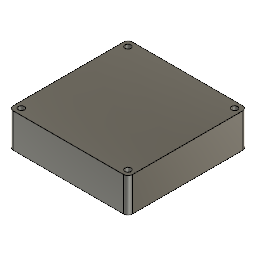
2024-12-28.2_development_hexapod_mounts (Autodesk Fusion 360 archive; units mm, degrees)
design "noctua_fan_80mm"
Autodesk Fusion 360 part; units mm, degrees
(part 1 of 2)
box "BoxPrimitive1" add length 80 width 80 height 23 placed x (0, -1, 0) y (1, 0, 0) z (0, 0, 1) at (0, 0, 0)
fillet "Fillet1" radius 3 4 edges at (0, -80, 11.5) (80, -80, 11.5) (80, 0, 11.5) (0, 0, 11.5)
sketch "Sketch2" plane through (0, 0, 23) normal (0, 0, 1) x (-1, 0, 0)
  arc A0 (-3, 0) -> (0, 3) centre (-3, 3) ccw
  line L0 (0, 3) -> (0, 77)
  arc A1 (0, 77) -> (-3, 80) centre (-3, 77) ccw
  line L1 (-3, 80) -> (-77, 80)
  arc A2 (-77, 80) -> (-80, 77) centre (-77, 77) ccw
  line L2 (-80, 77) -> (-80, 3)
  arc A3 (-80, 3) -> (-77, 0) centre (-77, 3) ccw
  line L3 (-77, 0) -> (-3, 0)
  circle A4 centre (-75.75, 75.75) radius 2
  circle A5 centre (-75.75, 4.25) radius 2
  circle A6 centre (-4.25, 75.75) radius 2
  circle A7 centre (-4.25, 4.25) radius 2
  dimension "d8" = 4
  dimension "d9" = 4
  dimension "d10" = 4
  dimension "d11" = 4
  dimension "d12" = 4.25
  dimension "d13" = 4.25
  dimension "d14" = 4.25
  dimension "d15" = 4.25
  dimension "d16" = 4.25
  dimension "d17" = 4.25
  dimension "d18" = 4.25
  dimension "d19" = 4.25
  measures "d8" diameter of A4
  measures "d9" diameter of A5
  measures "d10" diameter of A6
  measures "d11" diameter of A7
  measures "d12" distance of L1 A4.centre
  measures "d13" distance of L2 A4.centre
  measures "d14" distance of L3 A5.centre
  measures "d15" distance of L2 A5.centre
  measures "d16" distance of L3 A7.centre
  measures "d17" distance of L0 A7.centre
  measures "d18" distance of L1 A6.centre
  measures "d19" distance of L0 A6.centre
extrude "Extrude1" cut sketch "Sketch2" against normal blind 35 contours A4 | A5 | A6 | A7

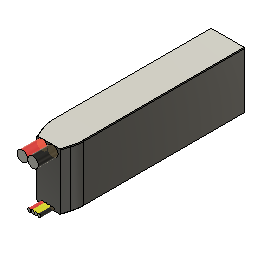
design "battery"
Autodesk Fusion 360 part; units mm, degrees
sketch "Sketch1" plane through (0, 0, 0) normal (0, 0, 1) x (1, 0, 0)
  line L0 (0, 0) -> (26, 0)
  line L1 (26, 0) -> (26, 137)
  line L2 (26, 137) -> (0, 137)
  line L3 (0, 137) -> (0, 0)
  dimension "d1" = 26
  dimension "d2" = 137
  constraint horizontal L0
  constraint vertical L1
  constraint horizontal L2
  constraint vertical L3
  constraint coincident L0.start L3.end
  measures "d1" distance of L0.start L0.end
  measures "d2" distance of L0.start L2.end
extrude "Extrude1" add sketch "Sketch1" along normal blind 43 makes body 1
sketch "Sketch2" plane through (0, 0, 0) normal (0, -1, 0) x (1, 0, 0)
  line L0 (0, 0) -> (26, 0)
  line L1 (26, 0) -> (26, 43)
  line L2 (26, 43) -> (0, 43)
  line L3 (0, 43) -> (0, 0)
  line L4 (21, 35) -> (5, 35) construction
  line L5 (5, 35) -> (5, 51) construction
  line L6 (5, 51) -> (21, 51) construction
  line L7 (21, 51) -> (21, 35) construction
  line L8 (21, 35) -> (5, 51) construction
  line L9 (5, 35) -> (21, 51) construction
  line L10 (13, 43) -> (5, 35) construction
  line L11 (13, 43) -> (21, 35) construction
  circle A0 centre (9, 39) radius 4
  circle A1 centre (17, 39) radius 4
  point P0 (13, 43)
  dimension "d5" = 16
  dimension "d6" = 16
  constraint horizontal L4
  constraint perpendicular L4 L5
  constraint parallel L4 L6
  constraint parallel L5 L7
  constraint coincident L8 P0
  constraint coincident L9 P0
  constraint midpoint L2 P0
  constraint coincident P0 L10.start
  constraint midpoint L10 A0.centre
  constraint tangent L2 A0
  constraint midpoint L11 A1.centre
  constraint tangent L2 A1
  measures "d5" distance of L5.end L6.end
  measures "d6" distance of L4.end L5.end
extrude "Extrude2" add sketch "Sketch2" along normal blind 15 separate body contours A0 | A1 makes body 2
sketch "Sketch3" plane through (0, 0, 0) normal (0, -1, 0) x (1, 0, 0)
  line L0 (0, 0) -> (26, 0)
  line L1 (26, 0) -> (26, 43)
  line L2 (26, 43) -> (0, 43)
  line L3 (0, 43) -> (0, 0)
  line L4 (18, 2.5) -> (8, 2.5) construction
  line L5 (8, 2.5) -> (8, -2.5) construction
  line L6 (8, -2.5) -> (18, -2.5) construction
  line L7 (18, -2.5) -> (18, 2.5) construction
  line L8 (18, 2.5) -> (8, -2.5) construction
  line L9 (8, 2.5) -> (18, -2.5) construction
  line L10 (8, 2.5) -> (8, 0)
  line L11 (8, 1.25) -> (9.25, 1.25) construction
  circle A0 centre (9.25, 1.25) radius 1.25
  circle A1 centre (11.75, 1.25) radius 1.25
  circle A2 centre (14.25, 1.25) radius 1.25
  circle A3 centre (16.75, 1.25) radius 1.25
  point P0 (13, 0)
  dimension "d9" = 10
  dimension "d10" = 5
  dimension "d11" = 1.25
  constraint horizontal L4
  constraint perpendicular L4 L5
  constraint parallel L4 L6
  constraint parallel L5 L7
  constraint coincident L8 P0
  constraint coincident L9 P0
  constraint midpoint L0 P0
  constraint midpoint L5 L10.end
  constraint midpoint L10 L11.start
  constraint perpendicular L5 L11
  constraint coincident L11.end A0.centre
  constraint tangent L4 A0
  measures "d9" distance of L5.end L6.end
  measures "d10" distance of L4.end L5.end
  measures "d11" distance of L11.start L11.end
extrude "Extrude3" add sketch "Sketch3" along normal blind 10 separate body contours A0 | A1 | A2 | A3 makes body 3
chamfer "Chamfer1" distance 3 distance2 10 1 edges at (26, 0, 21.5) measured on face at (8.6667, 0, 14.3333) on bodies 1
chamfer "Chamfer2" distance 12 distance2 5 1 edges at (0, 0, 21.5) measured on face at (0, 91.3333, 14.3333) on bodies 1
fillet "Fillet1" radius 30 2 edges at (0, 12, 21.5) (26, 10, 21.5) on bodies 1
chamfer "Chamfer3" distance 0.5 distance2 0.5 12 edges at (25.682, 10.0467, 0) (26, 75.7015, 0) (23.8674, 2.8913, 0) (0, 77.5, 0) (0.5826, 12.1165, 0) (3.6538, 3.2308, 0) (0.5826, 12.1165, 43) (0, 77.5, 43) (3.6538, 3.2308, 43) (26, 75.7015, 43) (23.8674, 2.8913, 43) (25.682, 10.0467, 43) 1 faces at (17.3333, 137, 14.3333) measured on face at (25.9843, 13.4317, 14.3333) measured on face at (26, 55.2687, 14.3333) measured on face at (23.5783, 1.9275, 14.3333) measured on face at (0, 97.3333, 14.3333) measured on face at (1.8284, 7.687, 28.6667) measured on face at (3.2051, 4.3077, 28.6667) measured on face at (1.8284, 7.687, 28.6667) measured on face at (17.3333, 56.4677, 43) measured on face at (3.2051, 4.3077, 28.6667) measured on face at (17.3333, 56.4677, 43) measured on face at (23.5783, 1.9275, 14.3333) measured on face at (25.9843, 13.4317, 14.3333) on bodies 1

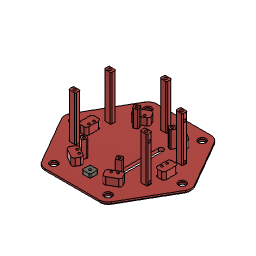
design "base"
Autodesk Fusion 360 part; units mm, degrees
sketch "Sketch1" plane through (0, 0, 0) normal (0, 0, 1) x (1, 0, 0)
  line L0 (130, 0) -> (65, 112.5833)
  line L1 (65, 112.5833) -> (-65, 112.5833)
  line L2 (-65, 112.5833) -> (-130, 0)
  line L3 (-130, 0) -> (-65, -112.5833)
  line L4 (-65, -112.5833) -> (65, -112.5833)
  line L5 (65, -112.5833) -> (130, 0)
  dimension "d1" = 130
  measures "d1" distance of L0.start origin
extrude "Extrude1" add sketch "Sketch1" along normal blind 6.5 makes body 1
fillet "Fillet1" radius 18 6 edges at (-130, 0, 3.25) (-65, -112.5833, 3.25) (65, -112.5833, 3.25) (130, 0, 3.25) (65, 112.5833, 3.25) (-65, 112.5833, 3.25) on bodies 1
chamfer "Chamfer2" distance 3.25 angle 45 12 edges at (0, -112.5833, 0) (63.6077, -110.1718, 0) (97.5, -56.2917, 0) (127.2154, 0, 0) (97.5, 56.2917, 0) (63.6077, 110.1718, 0) (0, 112.5833, 0) (-63.6077, 110.1718, 0) (-97.5, 56.2917, 0) (-127.2154, 0, 0) (-97.5, -56.2917, 0) (-63.6077, -110.1718, 0) on bodies 1
sketch "Sketch2" plane through (0, 0, 6.5) normal (0, 0, 1) x (-1, 0, 0)
  arc A0 (54.6077, -112.5833) -> (70.1962, -103.5833) centre (54.6077, -94.5833) ccw
  line L0 (70.1962, -103.5833) -> (124.8038, -9)
  arc A1 (124.8038, -9) -> (124.8038, 9) centre (109.2154, 0) ccw
  line L1 (124.8038, 9) -> (70.1962, 103.5833)
  line L2 (54.6077, 112.5833) -> (-54.6077, 112.5833)
  line L3 (-70.1962, 103.5833) -> (-124.8038, 9)
  arc A2 (-124.8038, 9) -> (-124.8038, -9) centre (-109.2154, 0) ccw
  line L4 (-124.8038, -9) -> (-70.1962, -103.5833)
  arc A3 (-70.1962, -103.5833) -> (-54.6077, -112.5833) centre (-54.6077, -94.5833) ccw
  line L5 (-54.6077, -112.5833) -> (54.6077, -112.5833)
  circle A4 centre (109.2154, 0) radius 7
  circle A5 centre (109.2154, 0) radius 6
  circle A6 centre (73.4654, -5) radius 2.25
  arc A7 (73.7154, 14.55) -> (68.7154, 9.55) centre (73.7154, 9.55) ccw
  line L6 (68.7154, 9.55) -> (68.7154, -9.55)
  circle A8 centre (73.4654, 5) radius 2.25
  line L7 (86.7154, 9.55) -> (86.7154, -9.55)
  line L8 (68.7154, 0) -> (86.7154, 0) construction
  arc A9 (68.7154, -9.55) -> (73.7154, -14.55) centre (73.7154, -9.55) ccw
  arc A10 (73.7154, 14.55) -> (68.7154, 9.55) centre (73.7154, 9.55) ccw
  line L9 (81.7154, 14.55) -> (73.7154, 14.55)
  line L10 (73.7154, -14.55) -> (81.7154, -14.55)
  line L11 (73.4654, 5) -> (68.7154, 5) construction
  line L12 (73.4654, -5) -> (68.7154, -5) construction
  line L13 (127.2154, 0) -> (-127.2154, 0) construction
  line L14 (0, -112.5833) -> (0, 112.5833) construction
  arc A11 (-124.8038, 9) -> (-124.8038, -9) centre (-109.2154, 0) ccw
  arc A12 (-70.1962, -103.5833) -> (-54.6077, -112.5833) centre (-54.6077, -94.5833) ccw
  arc A13 (54.6077, -112.5833) -> (70.1962, -103.5833) centre (54.6077, -94.5833) ccw
  arc A14 (81.7154, -14.55) -> (86.7154, -9.55) centre (81.7154, -9.55) ccw
  arc A15 (86.7154, 9.55) -> (81.7154, 14.55) centre (81.7154, 9.55) ccw
  circle A16 centre (32.4026, 66.1229) radius 2.25
  line L15 (34.3577, 59.5093) -> (43.3577, 75.0977) construction
  arc A17 (70.1962, 103.5833) -> (54.6077, 112.5833) centre (54.6077, 94.5833) ccw
  arc A18 (42.6282, 54.7343) -> (49.4584, 56.5644) centre (45.1282, 59.0644) ccw
  line L16 (41.0628, 61.1229) -> (38.6878, 57.0093) construction
  arc A19 (24.257, 71.1144) -> (26.0872, 64.2843) centre (28.5872, 68.6144) ccw
  line L17 (28.257, 78.0426) -> (24.257, 71.1144)
  circle A20 centre (41.0628, 61.1229) radius 2.25
  arc A21 (53.4584, 63.4926) -> (51.6282, 70.3227) centre (49.1282, 65.9926) ccw
  circle A22 centre (54.6077, 94.5833) radius 6
  circle A23 centre (54.6077, 94.5833) radius 7
  line L18 (32.4026, 66.1229) -> (30.0276, 62.0093) construction
  arc A24 (24.257, 71.1144) -> (26.0872, 64.2843) centre (28.5872, 68.6144) ccw
  line L19 (26.0872, 64.2843) -> (42.6282, 54.7343)
  line L20 (49.4584, 56.5644) -> (53.4584, 63.4926)
  line L21 (35.0872, 79.8727) -> (51.6282, 70.3227)
  arc A25 (35.0872, 79.8727) -> (28.257, 78.0426) centre (32.5872, 75.5426) ccw
  circle A26 centre (-41.0628, 61.1229) radius 2.25
  line L22 (-42.6282, 54.7343) -> (-26.0872, 64.2843)
  line L23 (-34.3577, 59.5093) -> (-43.3577, 75.0977) construction
  arc A27 (-54.6077, 112.5833) -> (-70.1962, 103.5833) centre (-54.6077, 94.5833) ccw
  arc A28 (-26.0872, 64.2843) -> (-24.257, 71.1144) centre (-28.5872, 68.6144) ccw
  line L24 (-32.4026, 66.1229) -> (-30.0276, 62.0093) construction
  arc A29 (-49.4584, 56.5644) -> (-42.6282, 54.7343) centre (-45.1282, 59.0644) ccw
  line L25 (-53.4584, 63.4926) -> (-49.4584, 56.5644)
  circle A30 centre (-32.4026, 66.1229) radius 2.25
  arc A31 (-28.257, 78.0426) -> (-35.0872, 79.8727) centre (-32.5872, 75.5426) ccw
  circle A32 centre (-54.6077, 94.5833) radius 6
  circle A33 centre (-54.6077, 94.5833) radius 7
  line L26 (-41.0628, 61.1229) -> (-38.6878, 57.0093) construction
  arc A34 (-49.4584, 56.5644) -> (-42.6282, 54.7343) centre (-45.1282, 59.0644) ccw
  line L27 (-42.6282, 54.7343) -> (-26.0872, 64.2843)
  line L28 (-24.257, 71.1144) -> (-28.257, 78.0426)
  line L29 (-51.6282, 70.3227) -> (-35.0872, 79.8727)
  arc A35 (-51.6282, 70.3227) -> (-53.4584, 63.4926) centre (-49.1282, 65.9926) ccw
  circle A36 centre (-73.4654, -5) radius 2.25
  line L30 (-68.7154, -9.55) -> (-68.7154, 9.55)
  line L31 (-68.7154, 0) -> (-86.7154, 0) construction
  arc A37 (-124.8038, 9) -> (-124.8038, -9) centre (-109.2154, 0) ccw
  arc A38 (-68.7154, 9.55) -> (-73.7154, 14.55) centre (-73.7154, 9.55) ccw
  line L32 (-73.4654, 5) -> (-68.7154, 5) construction
  arc A39 (-73.7154, -14.55) -> (-68.7154, -9.55) centre (-73.7154, -9.55) ccw
  line L33 (-81.7154, -14.55) -> (-73.7154, -14.55)
  circle A40 centre (-73.4654, 5) radius 2.25
  arc A41 (-81.7154, 14.55) -> (-86.7154, 9.55) centre (-81.7154, 9.55) ccw
  circle A42 centre (-109.2154, 0) radius 6
  circle A43 centre (-109.2154, 0) radius 7
  line L34 (-73.4654, -5) -> (-68.7154, -5) construction
  arc A44 (-73.7154, -14.55) -> (-68.7154, -9.55) centre (-73.7154, -9.55) ccw
  line L35 (-68.7154, -9.55) -> (-68.7154, 9.55)
  line L36 (-73.7154, 14.55) -> (-81.7154, 14.55)
  line L37 (-86.7154, -9.55) -> (-86.7154, 9.55)
  arc A45 (-86.7154, -9.55) -> (-81.7154, -14.55) centre (-81.7154, -9.55) ccw
  circle A46 centre (-32.4026, -66.1229) radius 2.25
  line L38 (-26.0872, -64.2843) -> (-42.6282, -54.7343)
  line L39 (-34.3577, -59.5093) -> (-43.3577, -75.0977) construction
  arc A47 (-70.1962, -103.5833) -> (-54.6077, -112.5833) centre (-54.6077, -94.5833) ccw
  arc A48 (-42.6282, -54.7343) -> (-49.4584, -56.5644) centre (-45.1282, -59.0644) ccw
  line L40 (-41.0628, -61.1229) -> (-38.6878, -57.0093) construction
  arc A49 (-24.257, -71.1144) -> (-26.0872, -64.2843) centre (-28.5872, -68.6144) ccw
  line L41 (-28.257, -78.0426) -> (-24.257, -71.1144)
  circle A50 centre (-41.0628, -61.1229) radius 2.25
  arc A51 (-53.4584, -63.4926) -> (-51.6282, -70.3227) centre (-49.1282, -65.9926) ccw
  circle A52 centre (-54.6077, -94.5833) radius 6
  circle A53 centre (-54.6077, -94.5833) radius 7
  line L42 (-32.4026, -66.1229) -> (-30.0276, -62.0093) construction
  arc A54 (-24.257, -71.1144) -> (-26.0872, -64.2843) centre (-28.5872, -68.6144) ccw
  line L43 (-26.0872, -64.2843) -> (-42.6282, -54.7343)
  line L44 (-49.4584, -56.5644) -> (-53.4584, -63.4926)
  line L45 (-35.0872, -79.8727) -> (-51.6282, -70.3227)
  arc A55 (-35.0872, -79.8727) -> (-28.257, -78.0426) centre (-32.5872, -75.5426) ccw
  circle A56 centre (41.0628, -61.1229) radius 2.25
  line L46 (34.3577, -59.5093) -> (43.3577, -75.0977) construction
  arc A57 (54.6077, -112.5833) -> (70.1962, -103.5833) centre (54.6077, -94.5833) ccw
  arc A58 (26.0872, -64.2843) -> (24.257, -71.1144) centre (28.5872, -68.6144) ccw
  line L47 (32.4026, -66.1229) -> (30.0276, -62.0093) construction
  arc A59 (49.4584, -56.5644) -> (42.6282, -54.7343) centre (45.1282, -59.0644) ccw
  line L48 (53.4584, -63.4926) -> (49.4584, -56.5644)
  circle A60 centre (32.4026, -66.1229) radius 2.25
  arc A61 (28.257, -78.0426) -> (35.0872, -79.8727) centre (32.5872, -75.5426) ccw
  circle A62 centre (54.6077, -94.5833) radius 6
  circle A63 centre (54.6077, -94.5833) radius 7
  line L49 (41.0628, -61.1229) -> (38.6878, -57.0093) construction
  arc A64 (49.4584, -56.5644) -> (42.6282, -54.7343) centre (45.1282, -59.0644) ccw
  line L50 (42.6282, -54.7343) -> (26.0872, -64.2843)
  line L51 (24.257, -71.1144) -> (28.257, -78.0426)
  line L52 (51.6282, -70.3227) -> (35.0872, -79.8727)
  arc A65 (51.6282, -70.3227) -> (53.4584, -63.4926) centre (49.1282, -65.9926) ccw
  circle A66 centre (73.4654, -5) radius 2.85
  circle A67 centre (73.4654, 5) radius 2.85
  circle A68 centre (41.0628, 61.1229) radius 2.85
  circle A69 centre (32.4026, 66.1229) radius 2.85
  circle A70 centre (-32.4026, 66.1229) radius 2.85
  circle A71 centre (-41.0628, 61.1229) radius 2.85
  circle A72 centre (-73.4654, 5) radius 2.85
  circle A73 centre (-73.4654, -5) radius 2.85
  circle A74 centre (-41.0628, -61.1229) radius 2.85
  circle A75 centre (-32.4026, -66.1229) radius 2.85
  circle A76 centre (32.4026, -66.1229) radius 2.85
  circle A77 centre (41.0628, -61.1229) radius 2.85
  line L53 (-77, -30.6738) -> (-67, -30.6738)
  line L54 (-65, -32.6738) -> (-65, -38.6134)
  line L55 (-67, -40.6134) -> (-77, -40.6134)
  line L56 (-79, -38.6134) -> (-79, -32.6738)
  line L57 (-77, 40.6096) -> (-67, 40.6096)
  line L58 (-65, 38.6096) -> (-65, 32.6738)
  line L59 (-67, 30.6738) -> (-77, 30.6738)
  line L60 (-79, 32.6738) -> (-79, 38.6096)
  line L61 (-72, -35.5) -> (-72, 13.37) construction
  line L62 (-72, 35.5) -> (-72, 30.8281) construction
  circle A78 centre (-72, 35.5) radius 2.85
  circle A79 centre (-72, -35.5) radius 2.85
  arc A80 (-65, -32.6738) -> (-67, -30.6738) centre (-67, -32.6738) ccw
  arc A81 (-67, -40.6134) -> (-65, -38.6134) centre (-67, -38.6134) ccw
  arc A82 (-77, -30.6738) -> (-79, -32.6738) centre (-77, -32.6738) ccw
  arc A83 (-79, -38.6134) -> (-77, -40.6134) centre (-77, -38.6134) ccw
  arc A84 (-67, 30.6738) -> (-65, 32.6738) centre (-67, 32.6738) ccw
  arc A85 (-65, 38.6096) -> (-67, 40.6096) centre (-67, 38.6096) ccw
  arc A86 (-77, 40.6096) -> (-79, 38.6096) centre (-77, 38.6096) ccw
  arc A87 (-79, 32.6738) -> (-77, 30.6738) centre (-77, 32.6738) ccw
  arc A88 (66.7634, -30.6879) -> (65, -32.6738) centre (67, -32.6738) ccw
  arc A89 (77, -40.6134) -> (79, -38.6134) centre (77, -38.6134) ccw
  line L63 (67, -40.6134) -> (77, -40.6134)
  arc A90 (79, -32.6738) -> (77, -30.6738) centre (77, -32.6738) ccw
  line L64 (79, -38.6134) -> (79, -32.6738)
  line L65 (65, -32.6738) -> (65, -38.6134)
  circle A91 centre (72, -35.5) radius 2.85
  arc A92 (65, -38.6134) -> (67, -40.6134) centre (67, -38.6134) ccw
  arc A93 (79, 38.6096) -> (77, 40.6096) centre (77, 38.6096) ccw
  line L66 (77, 40.6096) -> (67, 40.6096)
  arc A94 (77, 30.6738) -> (79, 32.6738) centre (77, 32.6738) ccw
  arc A95 (67, 40.6096) -> (65, 38.6096) centre (67, 38.6096) ccw
  circle A96 centre (72, 35.5) radius 2.85
  arc A97 (65, 32.6738) -> (66.7634, 30.6879) centre (67, 32.6738) ccw
  line L67 (-24, 37.5) -> (-24, -37.5)
  line L68 (-34, -37.5) -> (-34, 37.5)
  line L69 (-34, 40.2042) -> (-24, -40) construction
  line L70 (-24, 40) -> (-34, -40.2042) construction
  line L71 (68.7154, 0) -> (68.7154, 5) construction
  line L72 (63.7154, -5) -> (68.7154, 5) construction
  line L73 (68.7154, -5) -> (63.7154, 5) construction
  line L74 (-42.6282, -54.7343) -> (-26.0872, -64.2843)
  line L75 (42.6282, 54.7343) -> (26.0872, 64.2843)
  line L76 (-42.6282, 54.7343) -> (-26.0872, 64.2843)
  arc A98 (-34, -37.5) -> (-24, -37.5) centre (-29, -37.5) ccw
  arc A99 (-24, 37.5) -> (-34, 37.5) centre (-29, 37.5) ccw
  line L77 (-6, 84.2496) -> (6.5, 84.2496)
  line L78 (8.5, 82.2496) -> (8.5, 69.7496)
  line L79 (6.5, 67.7496) -> (-6, 67.7496)
  line L80 (-8, 69.7496) -> (-8, 82.2496)
  line L81 (-8, 84.2496) -> (8.5, 67.7496) construction
  line L82 (8.5, 84.2496) -> (-8, 67.7496) construction
  arc A100 (6.5, 67.7496) -> (8.5, 69.7496) centre (6.5, 69.7496) ccw
  arc A101 (8.5, 82.2496) -> (6.5, 84.2496) centre (6.5, 82.2496) ccw
  arc A102 (-6, 84.2496) -> (-8, 82.2496) centre (-6, 82.2496) ccw
  arc A103 (-8, 69.7496) -> (-6, 67.7496) centre (-6, 69.7496) ccw
  circle A104 centre (0.25, 75.9996) radius 2.25
  circle A105 centre (0.25, 75.9996) radius 2.85
  circle A106 centre (0, -76) radius 2.85
  line L83 (-5, -71) -> (5, -71)
  line L84 (7, -73) -> (7, -79)
  line L85 (5, -81) -> (-5, -81)
  line L86 (-7, -79) -> (-7, -73)
  line L87 (-7, -71) -> (7, -81) construction
  line L88 (7, -71) -> (-7, -81) construction
  arc A107 (5, -81) -> (7, -79) centre (5, -79) ccw
  arc A108 (7, -73) -> (5, -71) centre (5, -73) ccw
  arc A109 (-5, -71) -> (-7, -73) centre (-5, -73) ccw
  arc A110 (-7, -79) -> (-5, -81) centre (-5, -79) ccw
  line L89 (77, 30.6738) -> (66.7634, 30.6879)
  line L90 (77, -30.6738) -> (66.7634, -30.6879)
  line L91 (65, 32.6738) -> (65, 38.6096)
  line L92 (79, 32.6738) -> (79, 38.6096)
  line L93 (-35.8962, -47.074) -> (-30.7, -50.074)
  line L94 (-29.968, -52.8061) -> (-33.968, -59.7343)
  line L95 (-33.968, -59.7343) -> (-42.6282, -54.7343)
  line L96 (-42.6282, -54.7343) -> (-38.6282, -47.8061)
  line L97 (-37.6282, -46.074) -> (-33.968, -59.7343) construction
  line L98 (-28.968, -51.074) -> (-42.6282, -54.7343) construction
  line L99 (-24.257, -71.1144) -> (-16.5609, -57.7844) construction
  line L100 (-42.6282, -54.7343) -> (-38.8577, -48.2035) construction
  circle A111 centre (-35.7981, -52.9041) radius 2.25
  arc A112 (-29.968, -52.8061) -> (-30.7, -50.074) centre (-31.7, -51.8061) ccw
  arc A113 (-35.8962, -47.074) -> (-38.6282, -47.8061) centre (-36.8962, -48.8061) ccw
  line L101 (-29.968, 52.8061) -> (-33.968, 59.7343)
  line L102 (-35.8962, 47.074) -> (-30.7, 50.074)
  arc A114 (-30.7, 50.074) -> (-29.968, 52.8061) centre (-31.7, 51.8061) ccw
  arc A115 (-38.6282, 47.8061) -> (-35.8962, 47.074) centre (-36.8962, 48.8061) ccw
  line L103 (-42.6282, 54.7343) -> (-38.6282, 47.8061)
  circle A116 centre (-35.7981, 52.9041) radius 2.25
  line L104 (29.968, 52.8061) -> (33.968, 59.7343)
  arc A117 (29.968, 52.8061) -> (30.7, 50.074) centre (31.7, 51.8061) ccw
  line L105 (35.8962, 47.074) -> (30.7, 50.074)
  arc A118 (35.8962, 47.074) -> (38.6282, 47.8061) centre (36.8962, 48.8061) ccw
  line L106 (42.6282, 54.7343) -> (38.6282, 47.8061)
  circle A119 centre (35.7981, 52.9041) radius 2.25
  line L107 (29.968, -52.8061) -> (33.968, -59.7343)
  arc A120 (30.7, -50.074) -> (29.968, -52.8061) centre (31.7, -51.8061) ccw
  line L108 (35.8962, -47.074) -> (30.7, -50.074)
  arc A121 (38.6282, -47.8061) -> (35.8962, -47.074) centre (36.8962, -48.8061) ccw
  line L109 (42.6282, -54.7343) -> (38.6282, -47.8061)
  circle A122 centre (35.7981, -52.9041) radius 2.25
  point P0 (63.6077, 110.1718)
  point P1 (-63.6077, 110.1718)
  point P2 (-127.2154, 0)
  point P3 (-63.6077, -110.1718)
  point P4 (63.6077, -110.1718)
  point P5 (-72, -35.5)
  point P6 (-72, 35.5)
  point P7 (72, -35.5)
  point P8 (72, -35.5)
  point P9 (72, 35.5)
  point P10 (72, 35.5)
  point P11 (-28.9873, 0)
  point P12 (0, 76)
  point P13 (0, 72)
  point P14 (0.25, 75.9996)
  point P15 (0, -76)
  point P16 (-35.7981, -52.9041)
  point P17 (-35.7981, 52.9041)
  dimension "d8" = 14
  dimension "d9" = 12
  dimension "d10" = 18
  dimension "d11" = 9.55
  dimension "d12" = 9.55
  dimension "d15" = 29.1
  dimension "d30" = 5
  dimension "d33" = 4.5
  dimension "d34" = 4.5
  dimension "d35" = 5.7
  dimension "d36" = 5.7
  dimension "d49" = 72
  dimension "d50" = 5.7
  dimension "d51" = 5.7
  dimension "d53" = 2
  dimension "d75" = 35.5
  dimension "d76" = 35.5
  dimension "d78" = 80
  dimension "d79" = 24
  dimension "d84" = 5
  dimension "d85" = 5
  dimension "d86" = 10
  dimension "d135" = 10
  dimension "d164" = 16.5
  dimension "d165" = 16.5
  dimension "d166" = 2
  dimension "d170" = 76
  dimension "d171" = 4.5
  dimension "d172" = 5.7
  dimension "d173" = 5.7
  dimension "d174" = 76
  dimension "d175" = 14
  dimension "d176" = 10
  dimension "d177" = 2
  dimension "d188" = 7
  dimension "d189" = 7
  dimension "d190" = 10
  dimension "d191" = 10
  dimension "d192" = 4.5
  dimension "d193" = 2
  constraint concentric A1 A4
  constraint concentric A4 A5
  constraint coincident A7.end L6.start
  constraint coincident L6.end A9.start
  constraint coincident A9.end L10.start
  constraint coincident A7.start A10.start
  constraint coincident L8.end L7
  constraint parallel L9 L10
  constraint parallel L6 L7
  constraint coincident A8.centre L11.start
  constraint coincident A6.centre L12.start
  constraint midpoint A1 L13.start
  constraint midpoint A2 P2
  constraint midpoint L5 L14.start
  constraint midpoint L2 L14.end
  constraint collinear L8 L13
  constraint tangent L10 A14
  constraint tangent L7 A14
  constraint tangent L7 A15
  constraint tangent L9 A15
  constraint equal A14 A15
  constraint concentric A6 A66
  constraint horizontal L53
  constraint perpendicular L53 L54
  constraint parallel L53 L55
  constraint parallel L54 L56
  constraint horizontal L57
  constraint perpendicular L57 L58
  constraint parallel L57 L59
  constraint parallel L58 L60
  constraint coincident P5 L61.start
  constraint perpendicular L53 L61
  constraint coincident P6 L62.start
  constraint perpendicular L59 L62
  constraint collinear L61 L62
  constraint tangent L54 A80
  constraint tangent L53 A80
  constraint tangent L55 A81
  constraint tangent L54 A81
  constraint equal A80 A81
  constraint tangent L56 A82
  constraint tangent L53 A82
  constraint equal A80 A82
  constraint tangent L55 A83
  constraint tangent L56 A83
  constraint equal A80 A83
  constraint tangent L59 A84
  constraint tangent L58 A84
  constraint equal A80 A84
  constraint tangent L58 A85
  constraint tangent L57 A85
  constraint equal A80 A85
  constraint tangent L60 A86
  constraint tangent L57 A86
  constraint equal A80 A86
  constraint tangent L60 A87
  constraint tangent L59 A87
  constraint equal A80 A87
  constraint symmetric L14 P5 P8
  constraint symmetric L14 P6 P10
  constraint symmetric L14 A78 A96
  constraint symmetric L14 A79 A91
  constraint symmetric L14 L54.start A88.end
  constraint symmetric L14 A80 A88
  constraint symmetric L14 L55.start L63.start
  constraint symmetric L14 L54.end L65.end
  constraint symmetric L14 A81 A92
  constraint symmetric L14 L56.end A90.start
  constraint symmetric L14 L53.start A90.end
  constraint symmetric L14 A82 A90
  constraint symmetric L14 L55.end A89.start
  constraint symmetric L14 L56.start A89.end
  constraint symmetric L14 A83 A89
  constraint symmetric L14 L58.end A97.start
  constraint symmetric L14 A84 A97
  constraint symmetric L14 L58.start A95.end
  constraint symmetric L14 L57.end L66.end
  constraint symmetric L14 A85 A95
  constraint symmetric L14 L60.end A93.start
  constraint symmetric L14 L57.start A93.end
  constraint symmetric L14 A86 A93
  constraint symmetric L14 L60.start A94.end
  constraint symmetric L14 L59.end A94.start
  constraint symmetric L14 A87 A94
  constraint parallel L67 L68
  constraint coincident L69 P11
  constraint coincident L70 P11
  constraint coincident L13 P11
  constraint coincident L69.end L67
  constraint coincident L70.end L68
  constraint coincident L70.start L67
  constraint coincident L69.start L68
  constraint perpendicular L8 L71
  constraint symmetric L14 A58.start L38.start
  constraint symmetric L14 A59.end L38.end
  constraint symmetric L13 A58.start A19.end
  constraint symmetric L13 L38.start L22.end
  constraint tangent L68 A98
  constraint tangent L68 A99
  constraint horizontal L77
  constraint perpendicular L77 L78
  constraint parallel L77 L79
  constraint parallel L78 L80
  constraint coincident L81 P14
  constraint coincident L82 P14
  constraint coincident L81.end L79
  constraint coincident L81.end L78
  constraint tangent L79 A100
  constraint tangent L78 A100
  constraint coincident L82.start L78
  constraint coincident L82.start L77
  constraint tangent L78 A101
  constraint tangent L77 A101
  constraint equal A100 A101
  constraint coincident L81.start L77
  constraint coincident L81.start L80
  constraint tangent L77 A102
  constraint tangent L80 A102
  constraint equal A100 A102
  constraint coincident L82.end L80
  constraint coincident L82.end L79
  constraint tangent L80 A103
  constraint tangent L79 A103
  constraint equal A100 A103
  constraint coincident P14 A104.centre
  constraint concentric A104 A105
  constraint coincident L14 P15
  constraint horizontal L83
  constraint perpendicular L83 L84
  constraint parallel L83 L85
  constraint parallel L84 L86
  constraint coincident L87 P15
  constraint coincident L88 P15
  constraint coincident P15 A106.centre
  constraint coincident L87.end L85
  constraint coincident L87.end L84
  constraint tangent L85 A107
  constraint tangent L84 A107
  constraint coincident L88.start L84
  constraint coincident L88.start L83
  constraint tangent L84 A108
  constraint tangent L83 A108
  constraint equal A107 A108
  constraint coincident L87.start L83
  constraint coincident L87.start L86
  constraint tangent L83 A109
  constraint tangent L86 A109
  constraint equal A107 A109
  constraint coincident L88.end L86
  constraint coincident L88.end L85
  constraint tangent L86 A110
  constraint tangent L85 A110
  constraint equal A107 A110
  constraint tangent A93 L92
  constraint perpendicular L93 L94
  constraint parallel L93 L95
  constraint parallel L94 L96
  constraint coincident L97 P16
  constraint coincident L98 P16
  constraint collinear L43 L95
  constraint tangent A54 L99
  constraint parallel L41 L99
  constraint perpendicular L43 L100
  constraint collinear L96 L100
  constraint coincident P16 A111.centre
  constraint coincident L98.start L94
  constraint coincident L98.start L93
  constraint tangent L94 A112
  constraint tangent L93 A112
  constraint coincident L97.start L93
  constraint coincident L97.start L96
  constraint tangent L93 A113
  constraint tangent L96 A113
  constraint equal A112 A113
  constraint symmetric L13 L94.end L101.end
  constraint symmetric L13 L38.end L22.start
  constraint symmetric L13 P16 P17
  constraint symmetric L13 A111 A116
  constraint symmetric L13 L94.start L101.start
  constraint symmetric L13 L93.end L102.end
  constraint symmetric L13 A112 A114
  constraint symmetric L13 L93.start L102.start
  constraint symmetric L13 L96.end A115.start
  constraint symmetric L13 A113 A115
  constraint symmetric L14 L94.end L107.end
  constraint symmetric L14 L38.end A59.end
  constraint symmetric L14 A111 A122
  constraint symmetric L14 L94.start L107.start
  constraint symmetric L14 L93.end A120.start
  constraint symmetric L14 A112 A120
  constraint symmetric L14 L93.start L108.start
  constraint symmetric L14 L96.end A121.start
  constraint symmetric L14 A113 A121
  constraint symmetric L14 L101.start L104.start
  constraint symmetric L14 L101.end L104.end
  constraint symmetric L14 L102.start L105.start
  constraint symmetric L14 L102.end A117.end
  constraint symmetric L14 A114 A117
  constraint symmetric L14 A115.start A118.end
  constraint symmetric L14 A115 A118
  constraint symmetric L14 L22.start A18.start
  constraint symmetric L14 A116 A119
  measures "d8" diameter of A4
  measures "d9" diameter of A5
  measures "d10" distance of L8.end L8.start
  measures "d11" distance of A8.centre L9
  measures "d12" distance of A6.centre L10
  measures "d15" distance of L9 L10
  measures "d30" radius of A14
  measures "d33" diameter of A6
  measures "d34" diameter of A8
  measures "d35" diameter of A66
  measures "d36" diameter of A67
  measures "d49" distance of L14 P6
  measures "d50" diameter of A78
  measures "d51" diameter of A79
  measures "d53" radius of A80
  measures "d75" distance of L13 P5
  measures "d76" distance of L13 P6
  measures "d78" distance of L70.start L69.end
  measures "d79" distance of origin L67
  measures "d84" distance of L8.start L11.end
  measures "d85" distance of L11.end L73.end
  measures "d86" distance of L11.end L12.end
  measures "d135" distance of L67 L68
  measures "d164" distance of L81.end L82.end
  measures "d165" distance of L82.start L81.end
  measures "d166" radius of A100
  measures "d170" distance of origin P14
  measures "d171" diameter of A104
  measures "d172" diameter of A105
  measures "d173" diameter of A106
  measures "d174" distance of origin P15
  measures "d175" distance of L87.end L88.end
  measures "d176" distance of L88.start L87.end
  measures "d177" radius of A107
  measures "d188" distance of P8 L64
  measures "d189" distance of P8 L65
  measures "d190" distance of L94.end L38.end
  measures "d191" distance of L98.start L94.end
  measures "d192" diameter of A111
  measures "d193" radius of A112
extrude "Extrude2" cut sketch "Sketch2" against normal blind 6.5 contours A5 | A22 | A32 | A42 | A52 | A62 bodies 1
extrude "Extrude3" cut sketch "Sketch2" along normal blind 4.25 from surface at -6.5 contours A4 | A23 | A33 | A43 | A53 | A63 bodies 1
fillet "Fillet5" radius 0.5 6 edges at (-102.6891, 2.5313, 4.25) (-53.5367, -87.6657, 4.25) (49.1524, -90.197, 4.25) (-49.1524, 90.197, 4.25) (53.5367, 87.6657, 4.25) (102.6891, -2.5313, 4.25) on bodies 1
chamfer "Chamfer1" distance 1.5 angle 45 6 edges at (-103.6214, -2.1697, 6.5) (-53.6897, 88.6539, 6.5) (-49.9317, -90.8236, 6.5) (53.6897, -88.6539, 6.5) (49.9317, 90.8236, 6.5) (103.6214, 2.1697, 6.5) on bodies 1
extrude "Extrude4" add sketch "Sketch2" along normal blind 14.5 contours A7 L6 L7 A9 A10 L9 L10 A14 A15 | A18 A19 L17 A21 A24 L19 L20 L21 A25 L75 | L22 A28 A29 L25 A31 A34 L27 L28 L29 A35 L76 | L30 A38 A39 L33 A41 A44 L35 L36 L37 A45 | L38 A48 A49 L41 A51 A54 L43 L44 L45 A55 L74 L95 | A58 A59 L48 A61 A64 L50 L51 L52 A65 | A66 | A67 | A68 | A69 | A70 | A71 | A72 | A73 | A74 | A75 | A76 | A77 bodies 1
extrude "Extrude6" cut sketch "Sketch2" against normal blind 6.5 contours A6 | A8 | A16 | A20 | A26 | A30 | A36 | A40 | A46 | A50 | A56 | A60 | A66 | A67 | A68 | A69 | A70 | A71 | A72 | A73 | A74 | A75 | A76 | A77 bodies 1
extrude "Extrude25" add sketch "Sketch2" along normal blind 34 contours L19 L75 L104 A117 L105 A118 L106 | L22 L27 L76 L101 L102 A114 A115 L103 | L38 L43 L74 L93 L94 L95 L96 A112 A113 | L50 L107 A120 L108 A121 L109 | A111 | A116 | A119 | A122 bodies 1
extrude "Extrude26" cut sketch "Sketch2" against normal blind 5 from surface at 34 contours A111 | A116 | A119 | A122 bodies 1
extrude "Extrude7" add sketch "Sketch2" along normal blind 90 contours L53 L54 L55 L56 A80 A81 A82 A83 | L57 L58 L59 L60 A84 A85 A86 A87 | A78 | A79 | A88 A89 L63 A90 L64 L65 A92 L90 | A91 | A93 L66 A94 A95 A97 L89 L91 L92 | A96 | A106 | L83 L84 L85 L86 A107 A108 A109 A110 bodies 1
extrude "Extrude8" cut sketch "Sketch2" against normal blind 5 from surface at 90 contours A78 | A79 | A91 | A96 | A106 bodies 1
extrude "Extrude20" add sketch "Sketch2" along normal blind 7 separate body contours L77 L78 L79 L80 A100 A101 A102 A103 | A105 makes body 2
extrude "Extrude21" cut sketch "Sketch2" against normal blind 6.5 from surface at -1.5 contours A104 | A105 bodies 1
extrude "Extrude22" cut sketch "Sketch2" against normal blind 6.5 contours A104 bodies 1
sketch "Sketch4" plane through (79, 0, 0) normal (1, 0, 0) x (0, 1, 0)
  line L0 (32.6738, 6.5) -> (38.6134, 6.5)
  line L1 (38.6134, 6.5) -> (38.6134, 96.5)
  line L2 (38.6134, 96.5) -> (32.6738, 96.5)
  line L3 (32.6738, 96.5) -> (32.6738, 6.5)
  circle A0 centre (-35.6417, 82.5) radius 2.75
  circle A1 centre (-35.6417, 82.5) radius 1.75
  line L4 (-32.6738, 6.5) -> (-38.6096, 6.5) construction
  line L5 (38.6134, 6.5) -> (32.6738, 6.5) construction
  line L6 (-35.6417, 6.5) -> (-35.6417, 81) construction
  line L7 (-35.6417, 82.5) -> (-35.6417, 79.75) construction
  circle A2 centre (-35.6417, 10.5) radius 2.75
  circle A3 centre (-35.6417, 10.5) radius 1.75
  line L8 (0, 2.5) -> (0, 20) construction
  circle A4 centre (35.6417, 10.5) radius 1.75
  circle A5 centre (35.6417, 10.5) radius 2.75
  circle A6 centre (35.6417, 82.5) radius 1.75
  line L9 (35.6417, 6.5) -> (35.6417, 81) construction
  line L10 (32.6738, 6.5) -> (38.6096, 6.5) construction
  line L11 (35.6417, 82.5) -> (35.6417, 79.75) construction
  circle A7 centre (35.6417, 82.5) radius 2.75
  dimension "d59" = 5.5
  dimension "d60" = 3.5
  dimension "d62" = 76
  dimension "d63" = 5.5
  dimension "d64" = 4
  dimension "d65" = 3.5
  constraint concentric A0 A1
  constraint midpoint L4 L6.start
  constraint perpendicular L4 L6
  constraint coincident A0.centre A1.centre
  constraint coincident A0 L7.end
  constraint vertical L7
  constraint collinear L6 L7
  constraint coincident L6 A2.centre
  constraint concentric A2 A3
  constraint symmetric A0 L8 A7
  constraint symmetric A1 L8 A6
  constraint symmetric L4.start L8 L0.start
  constraint symmetric L4.end L8 L10.end
  constraint symmetric L6.start L8 L9.start
  constraint symmetric L6.end L8 L9.end
  constraint symmetric A0.centre L8 A6.centre
  constraint symmetric L7.end L8 L11.end
  constraint symmetric A2 L8 A5
  constraint symmetric A3 L8 A4
  measures "d59" diameter of A0
  measures "d60" diameter of A1
  measures "d62" distance of A0.centre L6.start
  measures "d63" diameter of A2
  measures "d64" distance of L4 A2.centre
  measures "d65" diameter of A3
extrude "Extrude9" cut sketch "Sketch4" against normal blind 5 contours A0 | A1 | A2 | A3 | A4 | A5 | A6 | A7 bodies 1
extrude "Extrude10" cut sketch "Sketch4" against normal up to surface (14 mm away) contours A1 | A3 | A4 | A6 bodies 1
extrude "Extrude11" cut sketch "Sketch2" against normal blind 6.5 contours L67 L68 A98 A99 bodies 1